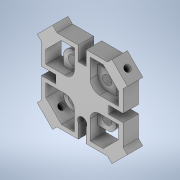
# Autodesk Inventor part: Interface Block
Saved by Autodesk Inventor 2022.2 (Build 262287010, 287A)
## iProperties
Created: 2022-02-02
Part Number: Interface Block
Material: ABS Plastic
Document SubType Name: Modeling
Designer: stmikutsky
Density: 1.06 g/cm^3
Appearance: Smooth - Medium Gray
Author: stmikutsky
Autodesk Inventor part; units mm, degrees
ref_plane "YZ Plane" through (0, 0, 0) normal (1, 0, 0) x (0, 1, 0)
ref_plane "XZ Plane" through (0, 0, 0) normal (0, 1, 0) x (-1, 0, 0)
ref_plane "XY Plane" through (0, 0, 0) normal (0, 0, 1) x (1, 0, 0)
sketch "Sketch1" plane through (0, 0, 0) normal (0, 0, 1) x (1, 0, 0)
  line L0 (-11.1369, 11.1369) -> (11.1369, 11.1369) construction
  line L1 (11.1369, 11.1369) -> (11.1369, -11.1369) construction
  line L2 (11.1369, -11.1369) -> (-11.1369, -11.1369) construction
  line L3 (-11.1369, -11.1369) -> (-11.1369, 11.1369) construction
  line L4 (-11.1369, 11.1369) -> (11.1369, -11.1369) construction
  line L5 (11.1369, 11.1369) -> (-11.1369, -11.1369) construction
  circle A0 centre (-11.1369, 11.1369) radius 3
  circle A1 centre (11.1369, 11.1369) radius 3
  circle A2 centre (-11.1369, -11.1369) radius 3
  circle A3 centre (0, -15.6056) radius 3
  circle A4 centre (11.1369, -11.1369) radius 3
  line L6 (-11.1369, -11.1369) -> (0, -15.6056) construction
  line L7 (0, -15.6056) -> (11.1369, -11.1369) construction
  line L8 (0, 0) -> (0, 30.7503) construction
  circle A5 centre (-11.1369, 11.1369) radius 6
  circle A6 centre (-11.1369, -11.1369) radius 6
  circle A7 centre (11.1369, -11.1369) radius 6
  circle A8 centre (11.1369, 11.1369) radius 6
  line L9 (-19.2384, -29.2384) -> (19.2384, -29.2384)
  line L10 (29.2384, -19.2384) -> (29.2384, 19.2384)
  line L11 (19.2384, 29.2384) -> (-19.2384, 29.2384)
  line L12 (-29.2384, 19.2384) -> (-29.2384, -19.2384)
  line L13 (-29.2384, -29.2384) -> (29.2384, 29.2384) construction
  line L14 (29.2384, -29.2384) -> (-29.2384, 29.2384) construction
  line L15 (-29.2384, 19.2384) -> (-19.2384, 29.2384)
  line L16 (19.2384, 29.2384) -> (29.2384, 19.2384)
  line L17 (29.2384, -19.2384) -> (19.2384, -29.2384)
  line L18 (-19.2384, -29.2384) -> (-29.2384, -19.2384)
  circle A9 centre (0, 0) radius 35 construction
  point P0 (0, 0)
  point P1 (25, 0)
  point P2 (0, 0)
  dimension "d31" = 70
  dimension "d2" = 31.5
  dimension "d4" = 6
  dimension "d5" = 6
  dimension "d6" = 12
  dimension "d18" = 12
  dimension "d21" = 10
  dimension "d22" = 10
  dimension "d23" = 10
  dimension "d24" = 10
  dimension "d25" = 10
  dimension "d26" = 10
  dimension "d27" = 10
  dimension "d28" = 10
  constraints: 38 end point, 10 coincident, 9 centre point, 9 point on line, 6 equal radius, 5 midpoint, 4 parallel, 2 equal length, 2 horizontal, 2 perpendicular, 1 vertical, 3 other
  measures "d2" distance of L0.start L1.end
  measures "d4" diameter of A3
  measures "d5" diameter of A4
  measures "d6" distance of L6.start L6.end
  measures "d18" diameter of A8
  measures "d21" distance of L12.start L14.end
  measures "d22" distance of L11.end L14.end
  measures "d23" distance of L11.start L13.end
  measures "d24" distance of L10.end L13.end
  measures "d25" distance of L10.start L14.start
  measures "d26" distance of L9.end L14.start
  measures "d27" distance of L9.start L13.start
  measures "d28" distance of L12.end L13.start
extrude "Extrusion1" add sketch "Sketch1" against normal blind 10 contours A5 | A6 | A7 | A8 | L18 L12 L15 L11 L16 L10 L17 L9
extrude "Extrusion3" cut sketch "Sketch1" against normal blind 5 contours A0 | A1 | A2 | A4 | A5 | A6 | A7 | A8
sketch "Sketch3" plane through (0, 0, 0) normal (0, 0, 1) x (1, 0, 0)
  circle A0 centre (-11.1369, -11.1369) radius 6 projected
  circle A1 centre (11.1369, -11.1369) radius 6 projected
  circle A2 centre (-11.1369, 11.1369) radius 6 projected
  circle A3 centre (11.1369, 11.1369) radius 6 projected
  line L0 (-29.2384, -19.2384) -> (-19.2384, -29.2384) projected
  line L1 (-19.2384, -29.2384) -> (19.2384, -29.2384) projected
  line L2 (19.2384, -29.2384) -> (29.2384, -19.2384) projected
  line L3 (29.2384, -19.2384) -> (29.2384, 19.2384) projected
  line L4 (29.2384, 19.2384) -> (19.2384, 29.2384) projected
  line L5 (19.2384, 29.2384) -> (-19.2384, 29.2384) projected
  line L6 (-19.2384, 29.2384) -> (-29.2384, 19.2384) projected
  line L7 (-29.2384, 19.2384) -> (-29.2384, -19.2384) projected
  circle A4 centre (0, -15.6056) radius 3 projected
  line L8 (19.2384, 29.2384) -> (16.41, 26.41)
  line L9 (13.5815, 23.5815) -> (23.5815, 13.5815)
  line L10 (23.5815, 13.5815) -> (26.41, 16.41) construction
  line L11 (29.2384, 19.2384) -> (29.2384, -19.2384) projected
  line L12 (29.2384, 19.2384) -> (19.2384, 29.2384) projected
  line L13 (23.5815, 13.5815) -> (23.5815, 5.1369)
  circle A5 centre (11.1369, 11.1369) radius 6 projected
  line L14 (26.41, 16.41) -> (26.41, 2.5685)
  line L15 (26.41, 16.41) -> (29.2384, 19.2384)
  line L16 (17.1369, 11.1369) -> (17.1369, 5.1369)
  line L17 (17.1369, 5.1369) -> (23.5815, 5.1369)
  line L18 (0, 0) -> (17.1369, 0) construction
  line L19 (16.41, 26.41) -> (2.5685, 26.41)
  line L20 (0, 17.1369) -> (0, 0) construction
  line L21 (16.41, 26.41) -> (13.5815, 23.5815) construction
  line L22 (13.5815, 23.5815) -> (5.1369, 23.5815)
  line L23 (5.1369, 23.5815) -> (5.1369, 17.1369)
  line L24 (5.1369, 17.1369) -> (11.1369, 17.1369)
  circle A6 centre (11.1369, 11.1369) radius 6 projected
  line L25 (0, 17.1369) -> (0, 29.2384)
  line L26 (19.2384, 29.2384) -> (-19.2384, 29.2384) projected
  line L27 (17.1369, 0) -> (29.2384, 0)
  line L28 (2.5685, 17.1369) -> (2.5685, 26.41)
  line L29 (0, 17.1369) -> (2.5685, 17.1369)
  line L30 (2.5685, 17.1369) -> (5.1369, 17.1369) construction
  line L31 (26.41, 2.5685) -> (17.1369, 2.5685)
  line L32 (17.1369, 2.5685) -> (17.1369, 0)
  line L33 (17.1369, 2.5685) -> (17.1369, 5.1369) construction
  dimension "d38" = 8
  constraints: 46 end point, 14 perpendicular, 6 horizontal, 5 collinear, 3 tangent, 3 vertical, 2 midpoint, 1 horizontal alignment, 1 point on circle, 1 other
  measures "d38" distance of L4.end L9.start
extrude "Extrusion5" cut sketch "Sketch3" against normal through all contours A3 L24 L23 L22 L9 L13 L17 L16 | L5 L8 L19 L28 L29 L25 | L27 L32 L31 L14 L15 L3
sketch "Sketch4" plane through (0, 0, -5) normal (0, 0, 1) x (1, 0, 0)
  circle A0 centre (11.1369, 11.1369) radius 3 projected
  arc A1 (11.1369, 17.1369) -> (17.1369, 11.1369) centre (11.1369, 11.1369) ccw projected
  arc A2 (17.1369, 11.1369) -> (11.1369, 17.1369) centre (11.1369, 11.1369) ccw projected
  line L0 (17.1369, 11.1369) -> (17.1369, 5.1369) projected
  line L1 (17.1369, 5.1369) -> (17.1369, 11.1369) projected
  line L2 (5.1369, 17.1369) -> (11.1369, 17.1369) projected
  line L3 (11.1369, 17.1369) -> (5.1369, 17.1369) projected
  line L4 (17.1369, 5.1369) -> (11.1369, 5.1369)
  line L5 (5.1369, 17.1369) -> (11.1369, 17.1369) projected
  line L6 (5.1369, 17.1369) -> (5.1369, 11.1369)
  point P0 (0, 0)
  constraints: 4 end point, 1 horizontal, 1 point on circle, 1 tangent
extrude "Extrusion6" cut sketch "Sketch4" along normal through all contours A1 L6 L2 | L0 L4 A1
pattern_circular "Circular Pattern2" count 4 over 360 about axis through (0, 0, -10) along (0, 0, 1) of "Extrusion5", "Extrusion6"
sketch "Sketch2" plane through (29.2384, 19.2384, -10) normal (0.7071, 0.7071, 0) x (-0.7071, 0.7071, 0)
  line L0 (0, 10) -> (0, 0) construction
  line L1 (14.1421, 0) -> (0, 0) construction
  line L2 (14.1421, 10) -> (14.1421, 0) construction
  line L3 (0, 10) -> (14.1421, 10) construction
  line L4 (14.1421, 10) -> (0, 0) construction
  circle A0 centre (7.0711, 5) radius 2
  point P0 (7.0711, 10)
  dimension "d32" = 4
  constraints: 2 end point, 1 centre point, 1 midpoint
  measures "d32" diameter of A0
extrude "Extrusion4" cut sketch "Sketch2" against normal up to next
pattern_circular "Circular Pattern1" count 4 over 360 about axis through (0, 0, -10) along (0, 0, 1) of "Extrusion4"
equation "\"d22\" = d21"
equation "\"d23\" = d21"
equation "\"d24\" = d23"
equation "\"d25\" = d21"
equation "\"d26\" = d25"
equation "\"d27\" = d21"
equation "\"d28\" = d27"
body "Solid1"
